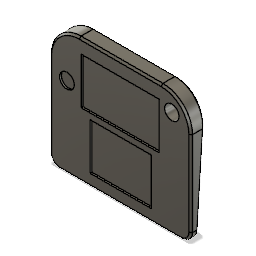
Key Chain - 2DS v1 (Autodesk Fusion 360 design; units mm, degrees)
Autodesk Fusion 360 part; units mm, degrees
note: some values were not read from the file. Set by a fixed rule: which sketch regions a step uses.
(part 1 of 2)
sketch "Sketch1" plane through (0, 0, 0) normal (0, 0, 1) x (1, 0, 0)
  line L0 (8.0698, -0.1323) -> (30.0302, -0.1323)
  arc A0 (30.0302, -0.1323) -> (37.9677, -8.0698) centre (30.0302, -8.0698) cw
  line L1 (37.9677, -8.0698) -> (37.9677, -30.824)
  arc A1 (37.9677, -30.824) -> (35.3219, -33.4698) centre (35.3219, -30.824) cw
  line L2 (35.3219, -33.4698) -> (2.7781, -33.4698)
  arc A2 (2.7781, -33.4698) -> (0.1323, -30.824) centre (2.7781, -30.824) cw
  line L3 (0.1323, -30.824) -> (0.1323, -8.0698)
  arc A3 (0.1323, -8.0698) -> (8.0698, -0.1323) centre (8.0698, -8.0698) cw
  line L4 (8.599, -3.8365) -> (29.501, -3.8365)
  line L5 (29.501, -3.8365) -> (29.501, -16.2719)
  line L6 (29.501, -16.2719) -> (8.599, -16.2719)
  line L7 (8.599, -16.2719) -> (8.599, -3.8365)
  circle A4 centre (4.7625, -11.9063) radius 1.9844
  line L8 (10.9802, -17.8594) -> (27.3844, -17.8594)
  line L9 (27.3844, -17.8594) -> (27.3844, -30.2948)
  line L10 (27.3844, -30.2948) -> (10.9802, -30.2948)
  line L11 (10.9802, -30.2948) -> (10.9802, -17.8594)
  point P0 (6.7469, -11.9063)
extrude "Extrude1" add sketch "Sketch1" along normal blind 2
extrude "Extrude2" add sketch "Sketch1" along normal blind 0.5 contours L4 L5 L6 L7 | A4 | L8 L9 L10 L11
scale "Scale1" factor 1.030792 about (37.9677, -8.0698, 2) bodies 1
draft "Draft1" angle 3.8 neutral plane through (35.2404, -34.2519, -0.0616) pull (0, -1, 0) 1 faces at (22.2403, -22.7972, -0.0616)
extrude "Extrude3" add 3 faces at (14.8765, -7.9789, 0.4538) (3.8617, -11.4913, 0.4538) (15.7856, -22.4336, 0.4538) along direction (0, 0, 1) blind 1.046
sketch "Sketch2" plane through (0, 0, 2) normal (0, 0, 1) x (1, 0, 0)
  circle A0 centre (3.7401, -12.0244) radius 2.0455
  line L0 (27.0585, -30.9791) -> (10.1492, -30.9791)
  line L1 (10.1492, -30.9791) -> (10.1492, -18.1608)
  line L2 (10.1492, -18.1608) -> (27.0585, -18.1608)
  line L3 (27.0585, -18.1608) -> (27.0585, -30.9791)
  line L4 (29.2403, -16.5244) -> (7.6946, -16.5244)
  line L5 (7.6946, -16.5244) -> (7.6946, -3.7061)
  line L6 (7.6946, -3.7061) -> (29.2403, -3.7061)
  line L7 (29.2403, -3.7061) -> (29.2403, -16.5244)
  line L8 (-1.0327, -8.0698) -> (-1.0327, -31.5246)
  arc A1 (-1.0327, -31.5246) -> (1.6946, -34.2519) centre (1.6946, -31.5246) ccw
  line L9 (1.6946, -34.2519) -> (35.2404, -34.2519)
  arc A2 (35.2404, -34.2519) -> (37.9677, -31.5246) centre (35.2404, -31.5246) ccw
  line L10 (37.9677, -31.5246) -> (37.9677, -8.0698)
  arc A3 (37.9677, -8.0698) -> (29.7858, 0.1121) centre (29.7858, -8.0698) ccw
  line L11 (29.7858, 0.1121) -> (7.1492, 0.1121)
  arc A4 (7.1492, 0.1121) -> (-1.0327, -8.0698) centre (7.1492, -8.0698) ccw
  line L12 (35.5713, -2.2843) -> (29.7858, -8.0698)
  line L13 (29.7858, -8.0698) -> (35.5713, -2.2843)
  line L14 (35.5713, -2.2843) -> (34.1571, -3.6985)
  circle A5 centre (32.7429, -5.1127) radius 2
  dimension "d10" = 2
  dimension "d11" = 4
  constraint midpoint A3 L12.start
  constraint coincident A3.centre L12.end
  constraint parallel L12 L13
  constraint parallel L13 L14
  constraint coincident L14.end A5
  measures "d10" distance of L12.start L14.end
  measures "d11" diameter of A5
extrude "Extrude4" cut sketch "Sketch2" against normal blind 27 contours L12 L13 A5 | L12 L13 A5
chamfer "Chamfer1" distance 0.5 angle 45 8 edges at (1.3637, -2.2843, 2) (-1.0327, -19.7972, 2) (-0.2339, -33.4531, 2) (18.4675, -34.2519, 2) (37.1689, -33.4531, 2) (37.9677, -19.7972, 2) (35.5713, -2.2843, 2) (18.4675, 0.1121, 2)
chamfer "Chamfer2" distance 0.5 angle 45 8 edges at (37.1689, -33.4531, -0.1146) (18.4675, -34.2519, -0.0616) (-0.2339, -33.4531, -0.1146) (-1.0327, -19.7972, -1.0217) (1.3637, -2.2843, -2.1849) (18.4675, 0.1121, -2.344) (35.5713, -2.2843, -2.1849) (37.9677, -19.7972, -1.0217)
sketch "Sketch3" plane through (0, -0.1545, -2.3263) normal (0, -0.066274, -0.997801) x (-1, 0, 0)
  ellipse E0 centre (-32.7429, -4.9691) end of major axis (-32.7429, -6.9736) minor radius 2
  spline S0 degree 3 poles (-7.1492, -0.2328) (-5.9064, -0.2328) (-4.6648, -0.5408) (-2.8861, -1.4812) (-2.2609, -1.9432) (-1.7176, -2.4877) (-1.1744, -3.0321) (-0.7133, -3.6587) (-0.0624, -4.8954) (0.1618, -5.487) (0.4582, -6.6971) (0.5327, -7.3149) (0.5327, -7.9327) knots -3.141593 -3.141593 -3.141593 -3.141593 -2.656195 -2.656195 -2.356194 -2.356194 -2.356194 -2.056194 -2.056194 -1.81147 -1.81147 -1.570796 -1.570796 -1.570796 -1.570796
  line L0 (-7.1492, -0.2328) -> (-29.7858, -0.2328)
  spline S1 degree 3 poles (-37.4677, -7.9327) (-37.4677, -6.6867) (-37.1602, -5.4418) (-36.2217, -3.6587) (-35.7606, -3.0321) (-35.2173, -2.4877) (-34.6741, -1.9432) (-34.0489, -1.4812) (-32.8198, -0.8314) (-32.2349, -0.608) (-31.0285, -0.3087) (-30.4072, -0.2328) (-29.7858, -0.2328) knots -1.570796 -1.570796 -1.570796 -1.570796 -1.085399 -1.085399 -0.785398 -0.785398 -0.785398 -0.485397 -0.485397 -0.242699 -0.242699 0 0 0 0
  line L1 (-37.4677, -7.9659) -> (-37.4677, -7.9327)
  line L2 (-37.4677, -7.9659) -> (-37.4677, -31.4392)
  spline S2 degree 3 poles (-37.4675, -31.4663) (-37.4676, -31.4618) (-37.4676, -31.4573) (-37.4677, -31.4482) (-37.4677, -31.4437) (-37.4677, -31.4392) knots -1.582946 -1.582946 -1.582946 -1.582946 -1.576871 -1.576871 -1.570796 -1.570796 -1.570796 -1.570796
  spline S3 degree 3 poles (-35.2404, -33.6725) (-35.6025, -33.6725) (-35.9643, -33.5823) (-36.4792, -33.3084) (-36.6588, -33.1753) (-36.815, -33.0188) (-36.9712, -32.8622) (-37.104, -32.6822) (-37.3733, -32.1737) (-37.4632, -31.8207) (-37.4675, -31.4663) knots -3.141593 -3.141593 -3.141593 -3.141593 -2.653648 -2.653648 -2.356194 -2.356194 -2.356194 -2.058741 -2.058741 -1.582946 -1.582946 -1.582946 -1.582946
  line L3 (-35.2404, -33.6725) -> (-1.6946, -33.6725)
  spline S4 degree 3 poles (0.5326, -31.4663) (0.5283, -31.8207) (0.4383, -32.1737) (0.169, -32.6822) (0.0362, -32.8622) (-0.12, -33.0188) (-0.2762, -33.1753) (-0.4558, -33.3084) (-0.9707, -33.5823) (-1.3325, -33.6725) (-1.6946, -33.6725) knots -1.558647 -1.558647 -1.558647 -1.558647 -1.082852 -1.082852 -0.785398 -0.785398 -0.785398 -0.487945 -0.487945 0 0 0 0
  spline S5 degree 3 poles (0.5327, -31.4392) (0.5327, -31.4437) (0.5327, -31.4482) (0.5327, -31.4573) (0.5326, -31.4618) (0.5326, -31.4663) knots -1.570796 -1.570796 -1.570796 -1.570796 -1.564722 -1.564722 -1.558647 -1.558647 -1.558647 -1.558647
  line L4 (0.5327, -31.4392) -> (0.5327, -7.9659)
  line L5 (0.5327, -7.9327) -> (0.5327, -7.9659)
  line L6 (-28.5549, -9.3081) -> (-28.5549, -9.5789)
  line L7 (-28.5549, -9.5789) -> (-28.8258, -9.5789)
  line L8 (-28.8258, -9.5789) -> (-28.8258, -9.8498)
  line L9 (-28.8258, -9.8498) -> (-29.0966, -9.8498)
  line L10 (-29.0966, -9.8498) -> (-29.0966, -10.1206)
  line L11 (-29.0966, -10.1206) -> (-29.3674, -10.1206)
  line L12 (-29.3674, -10.1206) -> (-29.3674, -10.3914)
  line L13 (-29.3674, -10.3914) -> (-29.6383, -10.3914)
  line L14 (-29.6383, -10.3914) -> (-29.6383, -10.6623)
  line L15 (-29.6383, -10.6623) -> (-29.9091, -10.6623)
  line L16 (-29.9091, -10.6623) -> (-29.9091, -11.2039)
  line L17 (-29.9091, -11.2039) -> (-28.2841, -11.2039)
  line L18 (-28.2841, -11.2039) -> (-28.2841, -15.2664)
  line L19 (-28.2841, -15.2664) -> (-29.9091, -15.2664)
  line L20 (-29.9091, -15.2664) -> (-29.9091, -16.6206)
  line L21 (-29.9091, -16.6206) -> (-25.8466, -16.6206)
  line L22 (-25.8466, -16.6206) -> (-25.8466, -15.2664)
  line L23 (-25.8466, -15.2664) -> (-26.9299, -15.2664)
  line L24 (-26.9299, -15.2664) -> (-26.9299, -9.3081)
  line L25 (-26.9299, -9.3081) -> (-28.5549, -9.3081)
  line L26 (-24.2216, -9.3081) -> (-24.2216, -9.5789)
  line L27 (-24.2216, -9.5789) -> (-24.4924, -9.5789)
  line L28 (-24.4924, -9.5789) -> (-24.4924, -9.8498)
  line L29 (-24.4924, -9.8498) -> (-24.7633, -9.8498)
  line L30 (-24.7633, -9.8498) -> (-24.7633, -10.1206)
  line L31 (-24.7633, -10.1206) -> (-25.0341, -10.1206)
  line L32 (-25.0341, -10.1206) -> (-25.0341, -10.3914)
  line L33 (-25.0341, -10.3914) -> (-25.3049, -10.3914)
  line L34 (-25.3049, -10.3914) -> (-25.3049, -15.5373)
  line L35 (-25.3049, -15.5373) -> (-25.0341, -15.5373)
  line L36 (-25.0341, -15.5373) -> (-25.0341, -15.8081)
  line L37 (-25.0341, -15.8081) -> (-24.7633, -15.8081)
  line L38 (-24.7633, -15.8081) -> (-24.7633, -16.0789)
  line L39 (-24.7633, -16.0789) -> (-24.4924, -16.0789)
  line L40 (-24.4924, -16.0789) -> (-24.4924, -16.3498)
  line L41 (-24.4924, -16.3498) -> (-24.2216, -16.3498)
  line L42 (-24.2216, -16.3498) -> (-24.2216, -16.6206)
  line L43 (-24.2216, -16.6206) -> (-21.7841, -16.6206)
  line L44 (-21.7841, -16.6206) -> (-21.7841, -16.3498)
  line L45 (-21.7841, -16.3498) -> (-21.5133, -16.3498)
  line L46 (-21.5133, -16.3498) -> (-21.5133, -16.0789)
  line L47 (-21.5133, -16.0789) -> (-21.2424, -16.0789)
  line L48 (-21.2424, -16.0789) -> (-21.2424, -15.8081)
  line L49 (-21.2424, -15.8081) -> (-20.9716, -15.8081)
  line L50 (-20.9716, -15.8081) -> (-20.9716, -13.3706)
  line L51 (-20.9716, -13.3706) -> (-21.2424, -13.3706)
  line L52 (-21.2424, -13.3706) -> (-21.2424, -13.0998)
  line L53 (-21.2424, -13.0998) -> (-21.5133, -13.0998)
  line L54 (-21.5133, -13.0998) -> (-21.5133, -12.8289)
  line L55 (-21.5133, -12.8289) -> (-21.7841, -12.8289)
  line L56 (-21.7841, -12.8289) -> (-21.7841, -12.5581)
  line L57 (-21.7841, -12.5581) -> (-22.0549, -12.5581)
  line L58 (-22.0549, -12.5581) -> (-22.0549, -12.2873)
  line L59 (-22.0549, -12.2873) -> (-23.6799, -12.2873)
  line L60 (-23.6799, -12.2873) -> (-23.6799, -12.5581)
  line L61 (-23.6799, -12.5581) -> (-23.9508, -12.5581)
  line L62 (-23.9508, -12.5581) -> (-23.9508, -11.4748)
  line L63 (-23.9508, -11.4748) -> (-23.6799, -11.4748)
  line L64 (-23.6799, -11.4748) -> (-23.6799, -11.2039)
  line L65 (-23.6799, -11.2039) -> (-23.4091, -11.2039)
  line L66 (-23.4091, -11.2039) -> (-23.4091, -10.9331)
  line L67 (-23.4091, -10.9331) -> (-22.5966, -10.9331)
  line L68 (-22.5966, -10.9331) -> (-22.5966, -11.2039)
  line L69 (-22.5966, -11.2039) -> (-22.3258, -11.2039)
  line L70 (-22.3258, -11.2039) -> (-22.3258, -11.7456)
  line L71 (-22.3258, -11.7456) -> (-20.9716, -11.7456)
  line L72 (-20.9716, -11.7456) -> (-20.9716, -10.3914)
  line L73 (-20.9716, -10.3914) -> (-21.2424, -10.3914)
  line L74 (-21.2424, -10.3914) -> (-21.2424, -10.1206)
  line L75 (-21.2424, -10.1206) -> (-21.5133, -10.1206)
  line L76 (-21.5133, -10.1206) -> (-21.5133, -9.8498)
  line L77 (-21.5133, -9.8498) -> (-21.7841, -9.8498)
  line L78 (-21.7841, -9.8498) -> (-21.7841, -9.5789)
  line L79 (-21.7841, -9.5789) -> (-22.0549, -9.5789)
  line L80 (-22.0549, -9.5789) -> (-22.0549, -9.3081)
  line L81 (-22.0549, -9.3081) -> (-24.2216, -9.3081)
  line L82 (-19.3466, -9.3081) -> (-19.3466, -16.6206)
  line L83 (-19.3466, -16.6206) -> (-16.9091, -16.6206)
  line L84 (-16.9091, -16.6206) -> (-16.9091, -16.3498)
  line L85 (-16.9091, -16.3498) -> (-16.6383, -16.3498)
  line L86 (-16.6383, -16.3498) -> (-16.6383, -16.0789)
  line L87 (-16.6383, -16.0789) -> (-16.3674, -16.0789)
  line L88 (-16.3674, -16.0789) -> (-16.3674, -15.8081)
  line L89 (-16.3674, -15.8081) -> (-16.0966, -15.8081)
  line L90 (-16.0966, -15.8081) -> (-16.0966, -13.3706)
  line L91 (-16.0966, -13.3706) -> (-16.3674, -13.3706)
  line L92 (-16.3674, -13.3706) -> (-16.3674, -13.0998)
  line L93 (-16.3674, -13.0998) -> (-16.6383, -13.0998)
  line L94 (-16.6383, -13.0998) -> (-16.6383, -12.8289)
  line L95 (-16.6383, -12.8289) -> (-16.3674, -12.8289)
  line L96 (-16.3674, -12.8289) -> (-16.3674, -12.5581)
  line L97 (-16.3674, -12.5581) -> (-16.0966, -12.5581)
  line L98 (-16.0966, -12.5581) -> (-16.0966, -10.1206)
  line L99 (-16.0966, -10.1206) -> (-16.3674, -10.1206)
  line L100 (-16.3674, -10.1206) -> (-16.3674, -9.8498)
  line L101 (-16.3674, -9.8498) -> (-16.6383, -9.8498)
  line L102 (-16.6383, -9.8498) -> (-16.6383, -9.5789)
  line L103 (-16.6383, -9.5789) -> (-16.9091, -9.5789)
  line L104 (-16.9091, -9.5789) -> (-16.9091, -9.3081)
  line L105 (-16.9091, -9.3081) -> (-19.3466, -9.3081)
  line L106 (-15.5549, -9.3081) -> (-15.5549, -10.6623)
  line L107 (-15.5549, -10.6623) -> (-14.4716, -10.6623)
  line L108 (-14.4716, -10.6623) -> (-14.4716, -15.2664)
  line L109 (-14.4716, -15.2664) -> (-15.5549, -15.2664)
  line L110 (-15.5549, -15.2664) -> (-15.5549, -16.6206)
  line L111 (-15.5549, -16.6206) -> (-11.7633, -16.6206)
  line L112 (-11.7633, -16.6206) -> (-11.7633, -15.2664)
  line L113 (-11.7633, -15.2664) -> (-12.8466, -15.2664)
  line L114 (-12.8466, -15.2664) -> (-12.8466, -10.6623)
  line L115 (-12.8466, -10.6623) -> (-11.7633, -10.6623)
  line L116 (-11.7633, -10.6623) -> (-11.7633, -9.3081)
  line L117 (-11.7633, -9.3081) -> (-15.5549, -9.3081)
  line L118 (-11.2216, -9.3081) -> (-11.2216, -10.6623)
  line L119 (-11.2216, -10.6623) -> (-10.1383, -10.6623)
  line L120 (-10.1383, -10.6623) -> (-10.1383, -16.6206)
  line L121 (-10.1383, -16.6206) -> (-8.5133, -16.6206)
  line L122 (-8.5133, -16.6206) -> (-8.5133, -10.6623)
  line L123 (-8.5133, -10.6623) -> (-7.4299, -10.6623)
  line L124 (-7.4299, -10.6623) -> (-7.4299, -9.3081)
  line L125 (-7.4299, -9.3081) -> (-11.2216, -9.3081)
  line L126 (-27.2008, -9.5789) -> (-27.2008, -15.5373)
  line L127 (-27.2008, -15.5373) -> (-26.1174, -15.5373)
  line L128 (-26.1174, -15.5373) -> (-26.1174, -16.3498)
  line L129 (-26.1174, -16.3498) -> (-29.6383, -16.3498)
  line L130 (-29.6383, -16.3498) -> (-29.6383, -15.5373)
  line L131 (-29.6383, -15.5373) -> (-28.0133, -15.5373)
  line L132 (-28.0133, -15.5373) -> (-28.0133, -10.9331)
  line L133 (-28.0133, -10.9331) -> (-29.3674, -10.9331)
  line L134 (-29.3674, -10.9331) -> (-29.3674, -10.6623)
  line L135 (-29.3674, -10.6623) -> (-29.0966, -10.6623)
  line L136 (-29.0966, -10.6623) -> (-29.0966, -10.3914)
  line L137 (-29.0966, -10.3914) -> (-28.8258, -10.3914)
  line L138 (-28.8258, -10.3914) -> (-28.8258, -10.1206)
  line L139 (-28.8258, -10.1206) -> (-28.5549, -10.1206)
  line L140 (-28.5549, -10.1206) -> (-28.5549, -9.8498)
  line L141 (-28.5549, -9.8498) -> (-28.2841, -9.8498)
  line L142 (-28.2841, -9.8498) -> (-28.2841, -9.5789)
  line L143 (-28.2841, -9.5789) -> (-27.2008, -9.5789)
  line L144 (-22.3258, -9.5789) -> (-22.3258, -9.8498)
  line L145 (-22.3258, -9.8498) -> (-22.0549, -9.8498)
  line L146 (-22.0549, -9.8498) -> (-22.0549, -10.1206)
  line L147 (-22.0549, -10.1206) -> (-21.7841, -10.1206)
  line L148 (-21.7841, -10.1206) -> (-21.7841, -10.3914)
  line L149 (-21.7841, -10.3914) -> (-21.5133, -10.3914)
  line L150 (-21.5133, -10.3914) -> (-21.5133, -10.6623)
  line L151 (-21.5133, -10.6623) -> (-21.2424, -10.6623)
  line L152 (-21.2424, -10.6623) -> (-21.2424, -11.4748)
  line L153 (-21.2424, -11.4748) -> (-22.0549, -11.4748)
  line L154 (-22.0549, -11.4748) -> (-22.0549, -10.9331)
  line L155 (-22.0549, -10.9331) -> (-22.3258, -10.9331)
  line L156 (-22.3258, -10.9331) -> (-22.3258, -10.6623)
  line L157 (-22.3258, -10.6623) -> (-23.6799, -10.6623)
  line L158 (-23.6799, -10.6623) -> (-23.6799, -10.9331)
  line L159 (-23.6799, -10.9331) -> (-23.9508, -10.9331)
  line L160 (-23.9508, -10.9331) -> (-23.9508, -11.2039)
  line L161 (-23.9508, -11.2039) -> (-24.2216, -11.2039)
  line L162 (-24.2216, -11.2039) -> (-24.2216, -13.0998)
  line L163 (-24.2216, -13.0998) -> (-23.6799, -13.0998)
  line L164 (-23.6799, -13.0998) -> (-23.6799, -12.8289)
  line L165 (-23.6799, -12.8289) -> (-23.4091, -12.8289)
  line L166 (-23.4091, -12.8289) -> (-23.4091, -12.5581)
  line L167 (-23.4091, -12.5581) -> (-22.3258, -12.5581)
  line L168 (-22.3258, -12.5581) -> (-22.3258, -12.8289)
  line L169 (-22.3258, -12.8289) -> (-22.0549, -12.8289)
  line L170 (-22.0549, -12.8289) -> (-22.0549, -13.0998)
  line L171 (-22.0549, -13.0998) -> (-21.7841, -13.0998)
  line L172 (-21.7841, -13.0998) -> (-21.7841, -13.3706)
  line L173 (-21.7841, -13.3706) -> (-21.5133, -13.3706)
  line L174 (-21.5133, -13.3706) -> (-21.5133, -13.6414)
  line L175 (-21.5133, -13.6414) -> (-21.2424, -13.6414)
  line L176 (-21.2424, -13.6414) -> (-21.2424, -15.5373)
  line L177 (-21.2424, -15.5373) -> (-21.5133, -15.5373)
  line L178 (-21.5133, -15.5373) -> (-21.5133, -15.8081)
  line L179 (-21.5133, -15.8081) -> (-21.7841, -15.8081)
  line L180 (-21.7841, -15.8081) -> (-21.7841, -16.0789)
  line L181 (-21.7841, -16.0789) -> (-22.0549, -16.0789)
  line L182 (-22.0549, -16.0789) -> (-22.0549, -16.3498)
  line L183 (-22.0549, -16.3498) -> (-23.9508, -16.3498)
  line L184 (-23.9508, -16.3498) -> (-23.9508, -16.0789)
  line L185 (-23.9508, -16.0789) -> (-24.2216, -16.0789)
  line L186 (-24.2216, -16.0789) -> (-24.2216, -15.8081)
  line L187 (-24.2216, -15.8081) -> (-24.4924, -15.8081)
  line L188 (-24.4924, -15.8081) -> (-24.4924, -15.5373)
  line L189 (-24.4924, -15.5373) -> (-24.7633, -15.5373)
  line L190 (-24.7633, -15.5373) -> (-24.7633, -15.2664)
  line L191 (-24.7633, -15.2664) -> (-25.0341, -15.2664)
  line L192 (-25.0341, -15.2664) -> (-25.0341, -10.6623)
  line L193 (-25.0341, -10.6623) -> (-24.7633, -10.6623)
  line L194 (-24.7633, -10.6623) -> (-24.7633, -10.3914)
  line L195 (-24.7633, -10.3914) -> (-24.4924, -10.3914)
  line L196 (-24.4924, -10.3914) -> (-24.4924, -10.1206)
  line L197 (-24.4924, -10.1206) -> (-24.2216, -10.1206)
  line L198 (-24.2216, -10.1206) -> (-24.2216, -9.8498)
  line L199 (-24.2216, -9.8498) -> (-23.9508, -9.8498)
  line L200 (-23.9508, -9.8498) -> (-23.9508, -9.5789)
  line L201 (-23.9508, -9.5789) -> (-22.3258, -9.5789)
  line L202 (-17.1799, -9.5789) -> (-17.1799, -9.8498)
  line L203 (-17.1799, -9.8498) -> (-16.9091, -9.8498)
  line L204 (-16.9091, -9.8498) -> (-16.9091, -10.1206)
  line L205 (-16.9091, -10.1206) -> (-16.6383, -10.1206)
  line L206 (-16.6383, -10.1206) -> (-16.6383, -10.3914)
  line L207 (-16.6383, -10.3914) -> (-16.3674, -10.3914)
  line L208 (-16.3674, -10.3914) -> (-16.3674, -12.2873)
  line L209 (-16.3674, -12.2873) -> (-16.6383, -12.2873)
  line L210 (-16.6383, -12.2873) -> (-16.6383, -12.5581)
  line L211 (-16.6383, -12.5581) -> (-17.4508, -12.5581)
  line L212 (-17.4508, -12.5581) -> (-17.4508, -12.8289)
  line L213 (-17.4508, -12.8289) -> (-17.1799, -12.8289)
  line L214 (-17.1799, -12.8289) -> (-17.1799, -13.0998)
  line L215 (-17.1799, -13.0998) -> (-16.9091, -13.0998)
  line L216 (-16.9091, -13.0998) -> (-16.9091, -13.3706)
  line L217 (-16.9091, -13.3706) -> (-16.6383, -13.3706)
  line L218 (-16.6383, -13.3706) -> (-16.6383, -13.6414)
  line L219 (-16.6383, -13.6414) -> (-16.3674, -13.6414)
  line L220 (-16.3674, -13.6414) -> (-16.3674, -15.5373)
  line L221 (-16.3674, -15.5373) -> (-16.6383, -15.5373)
  line L222 (-16.6383, -15.5373) -> (-16.6383, -15.8081)
  line L223 (-16.6383, -15.8081) -> (-16.9091, -15.8081)
  line L224 (-16.9091, -15.8081) -> (-16.9091, -16.0789)
  line L225 (-16.9091, -16.0789) -> (-17.1799, -16.0789)
  line L226 (-17.1799, -16.0789) -> (-17.1799, -16.3498)
  line L227 (-17.1799, -16.3498) -> (-19.0758, -16.3498)
  line L228 (-19.0758, -16.3498) -> (-19.0758, -9.5789)
  line L229 (-19.0758, -9.5789) -> (-17.1799, -9.5789)
  line L230 (-12.0341, -9.5789) -> (-12.0341, -10.3914)
  line L231 (-12.0341, -10.3914) -> (-13.1174, -10.3914)
  line L232 (-13.1174, -10.3914) -> (-13.1174, -15.5373)
  line L233 (-13.1174, -15.5373) -> (-12.0341, -15.5373)
  line L234 (-12.0341, -15.5373) -> (-12.0341, -16.3498)
  line L235 (-12.0341, -16.3498) -> (-15.2841, -16.3498)
  line L236 (-15.2841, -16.3498) -> (-15.2841, -15.5373)
  line L237 (-15.2841, -15.5373) -> (-14.2008, -15.5373)
  line L238 (-14.2008, -15.5373) -> (-14.2008, -10.3914)
  line L239 (-14.2008, -10.3914) -> (-15.2841, -10.3914)
  line L240 (-15.2841, -10.3914) -> (-15.2841, -9.5789)
  line L241 (-15.2841, -9.5789) -> (-12.0341, -9.5789)
  line L242 (-7.7008, -9.5789) -> (-7.7008, -10.3914)
  line L243 (-7.7008, -10.3914) -> (-8.7841, -10.3914)
  line L244 (-8.7841, -10.3914) -> (-8.7841, -16.3498)
  line L245 (-8.7841, -16.3498) -> (-9.8674, -16.3498)
  line L246 (-9.8674, -16.3498) -> (-9.8674, -10.3914)
  line L247 (-9.8674, -10.3914) -> (-10.9508, -10.3914)
  line L248 (-10.9508, -10.3914) -> (-10.9508, -9.5789)
  line L249 (-10.9508, -9.5789) -> (-7.7008, -9.5789)
  line L250 (-18.5341, -10.1206) -> (-18.5341, -12.0164)
  line L251 (-18.5341, -12.0164) -> (-17.4508, -12.0164)
  line L252 (-17.4508, -12.0164) -> (-17.4508, -11.7456)
  line L253 (-17.4508, -11.7456) -> (-17.1799, -11.7456)
  line L254 (-17.1799, -11.7456) -> (-17.1799, -10.3914)
  line L255 (-17.1799, -10.3914) -> (-17.4508, -10.3914)
  line L256 (-17.4508, -10.3914) -> (-17.4508, -10.1206)
  line L257 (-17.4508, -10.1206) -> (-18.5341, -10.1206)
  line L258 (-17.7216, -10.3914) -> (-17.7216, -10.6623)
  line L259 (-17.7216, -10.6623) -> (-17.4508, -10.6623)
  line L260 (-17.4508, -10.6623) -> (-17.4508, -11.4748)
  line L261 (-17.4508, -11.4748) -> (-17.7216, -11.4748)
  line L262 (-17.7216, -11.4748) -> (-17.7216, -11.7456)
  line L263 (-17.7216, -11.7456) -> (-18.2633, -11.7456)
  line L264 (-18.2633, -11.7456) -> (-18.2633, -10.3914)
  line L265 (-18.2633, -10.3914) -> (-17.7216, -10.3914)
  line L266 (-23.6799, -13.3706) -> (-23.6799, -13.6414)
  line L267 (-23.6799, -13.6414) -> (-23.9508, -13.6414)
  line L268 (-23.9508, -13.6414) -> (-23.9508, -13.9123)
  line L269 (-23.9508, -13.9123) -> (-24.2216, -13.9123)
  line L270 (-24.2216, -13.9123) -> (-24.2216, -15.2664)
  line L271 (-24.2216, -15.2664) -> (-23.9508, -15.2664)
  line L272 (-23.9508, -15.2664) -> (-23.9508, -15.5373)
  line L273 (-23.9508, -15.5373) -> (-23.6799, -15.5373)
  line L274 (-23.6799, -15.5373) -> (-23.6799, -15.8081)
  line L275 (-23.6799, -15.8081) -> (-22.5966, -15.8081)
  line L276 (-22.5966, -15.8081) -> (-22.5966, -15.5373)
  line L277 (-22.5966, -15.5373) -> (-22.3258, -15.5373)
  line L278 (-22.3258, -15.5373) -> (-22.3258, -15.2664)
  line L279 (-22.3258, -15.2664) -> (-22.0549, -15.2664)
  line L280 (-22.0549, -15.2664) -> (-22.0549, -13.9123)
  line L281 (-22.0549, -13.9123) -> (-22.3258, -13.9123)
  line L282 (-22.3258, -13.9123) -> (-22.3258, -13.6414)
  line L283 (-22.3258, -13.6414) -> (-22.5966, -13.6414)
  line L284 (-22.5966, -13.6414) -> (-22.5966, -13.3706)
  line L285 (-22.5966, -13.3706) -> (-23.6799, -13.3706)
  line L286 (-18.5341, -13.3706) -> (-18.5341, -15.5373)
  line L287 (-18.5341, -15.5373) -> (-17.4508, -15.5373)
  line L288 (-17.4508, -15.5373) -> (-17.4508, -15.2664)
  line L289 (-17.4508, -15.2664) -> (-17.1799, -15.2664)
  line L290 (-17.1799, -15.2664) -> (-17.1799, -13.6414)
  line L291 (-17.1799, -13.6414) -> (-17.4508, -13.6414)
  line L292 (-17.4508, -13.6414) -> (-17.4508, -13.3706)
  line L293 (-17.4508, -13.3706) -> (-18.5341, -13.3706)
  line L294 (-22.8674, -13.6414) -> (-22.8674, -13.9123)
  line L295 (-22.8674, -13.9123) -> (-22.5966, -13.9123)
  line L296 (-22.5966, -13.9123) -> (-22.5966, -14.1831)
  line L297 (-22.5966, -14.1831) -> (-22.3258, -14.1831)
  line L298 (-22.3258, -14.1831) -> (-22.3258, -14.9956)
  line L299 (-22.3258, -14.9956) -> (-22.5966, -14.9956)
  line L300 (-22.5966, -14.9956) -> (-22.5966, -15.2664)
  line L301 (-22.5966, -15.2664) -> (-22.8674, -15.2664)
  line L302 (-22.8674, -15.2664) -> (-22.8674, -15.5373)
  line L303 (-22.8674, -15.5373) -> (-23.4091, -15.5373)
  line L304 (-23.4091, -15.5373) -> (-23.4091, -15.2664)
  line L305 (-23.4091, -15.2664) -> (-23.6799, -15.2664)
  line L306 (-23.6799, -15.2664) -> (-23.6799, -14.9956)
  line L307 (-23.6799, -14.9956) -> (-23.9508, -14.9956)
  line L308 (-23.9508, -14.9956) -> (-23.9508, -14.1831)
  line L309 (-23.9508, -14.1831) -> (-23.6799, -14.1831)
  line L310 (-23.6799, -14.1831) -> (-23.6799, -13.9123)
  line L311 (-23.6799, -13.9123) -> (-23.4091, -13.9123)
  line L312 (-23.4091, -13.9123) -> (-23.4091, -13.6414)
  line L313 (-23.4091, -13.6414) -> (-22.8674, -13.6414)
  line L314 (-17.7216, -13.6414) -> (-17.7216, -13.9123)
  line L315 (-17.7216, -13.9123) -> (-17.4508, -13.9123)
  line L316 (-17.4508, -13.9123) -> (-17.4508, -14.9956)
  line L317 (-17.4508, -14.9956) -> (-17.7216, -14.9956)
  line L318 (-17.7216, -14.9956) -> (-17.7216, -15.2664)
  line L319 (-17.7216, -15.2664) -> (-18.2633, -15.2664)
  line L320 (-18.2633, -15.2664) -> (-18.2633, -13.6414)
  line L321 (-18.2633, -13.6414) -> (-17.7216, -13.6414)
  line L322 (-28.8258, -17.4331) -> (-28.8258, -17.7039)
  line L323 (-28.8258, -17.7039) -> (-29.0966, -17.7039)
  line L324 (-29.0966, -17.7039) -> (-29.0966, -17.9748)
  line L325 (-29.0966, -17.9748) -> (-29.3674, -17.9748)
  line L326 (-29.3674, -17.9748) -> (-29.3674, -18.2456)
  line L327 (-29.3674, -18.2456) -> (-29.6383, -18.2456)
  line L328 (-29.6383, -18.2456) -> (-29.6383, -18.5164)
  line L329 (-29.6383, -18.5164) -> (-29.9091, -18.5164)
  line L330 (-29.9091, -18.5164) -> (-29.9091, -21.2248)
  line L331 (-29.9091, -21.2248) -> (-29.6383, -21.2248)
  line L332 (-29.6383, -21.2248) -> (-29.6383, -21.4956)
  line L333 (-29.6383, -21.4956) -> (-29.3674, -21.4956)
  line L334 (-29.3674, -21.4956) -> (-29.3674, -21.7664)
  line L335 (-29.3674, -21.7664) -> (-29.0966, -21.7664)
  line L336 (-29.0966, -21.7664) -> (-29.0966, -22.0373)
  line L337 (-29.0966, -22.0373) -> (-28.8258, -22.0373)
  line L338 (-28.8258, -22.0373) -> (-28.8258, -22.3081)
  line L339 (-28.8258, -22.3081) -> (-26.9299, -22.3081)
  line L340 (-26.9299, -22.3081) -> (-26.9299, -22.0373)
  line L341 (-26.9299, -22.0373) -> (-26.6591, -22.0373)
  line L342 (-26.6591, -22.0373) -> (-26.6591, -21.7664)
  line L343 (-26.6591, -21.7664) -> (-26.3883, -21.7664)
  line L344 (-26.3883, -21.7664) -> (-26.3883, -21.4956)
  line L345 (-26.3883, -21.4956) -> (-26.1174, -21.4956)
  line L346 (-26.1174, -21.4956) -> (-26.1174, -19.3289)
  line L347 (-26.1174, -19.3289) -> (-28.0133, -19.3289)
  line L348 (-28.0133, -19.3289) -> (-28.0133, -20.4123)
  line L349 (-28.0133, -20.4123) -> (-26.9299, -20.4123)
  line L350 (-26.9299, -20.4123) -> (-26.9299, -20.6831)
  line L351 (-26.9299, -20.6831) -> (-27.2008, -20.6831)
  line L352 (-27.2008, -20.6831) -> (-27.2008, -20.9539)
  line L353 (-27.2008, -20.9539) -> (-27.4716, -20.9539)
  line L354 (-27.4716, -20.9539) -> (-27.4716, -21.2248)
  line L355 (-27.4716, -21.2248) -> (-28.2841, -21.2248)
  line L356 (-28.2841, -21.2248) -> (-28.2841, -20.9539)
  line L357 (-28.2841, -20.9539) -> (-28.5549, -20.9539)
  line L358 (-28.5549, -20.9539) -> (-28.5549, -20.6831)
  line L359 (-28.5549, -20.6831) -> (-28.8258, -20.6831)
  line L360 (-28.8258, -20.6831) -> (-28.8258, -19.0581)
  line L361 (-28.8258, -19.0581) -> (-28.5549, -19.0581)
  line L362 (-28.5549, -19.0581) -> (-28.5549, -18.7873)
  line L363 (-28.5549, -18.7873) -> (-28.2841, -18.7873)
  line L364 (-28.2841, -18.7873) -> (-28.2841, -18.5164)
  line L365 (-28.2841, -18.5164) -> (-26.9299, -18.5164)
  line L366 (-26.9299, -18.5164) -> (-26.9299, -17.4331)
  line L367 (-26.9299, -17.4331) -> (-28.8258, -17.4331)
  line L368 (-23.9508, -17.4331) -> (-23.9508, -17.7039)
  line L369 (-23.9508, -17.7039) -> (-24.2216, -17.7039)
  line L370 (-24.2216, -17.7039) -> (-24.2216, -17.9748)
  line L371 (-24.2216, -17.9748) -> (-24.4924, -17.9748)
  line L372 (-24.4924, -17.9748) -> (-24.4924, -18.2456)
  line L373 (-24.4924, -18.2456) -> (-24.7633, -18.2456)
  line L374 (-24.7633, -18.2456) -> (-24.7633, -18.5164)
  line L375 (-24.7633, -18.5164) -> (-25.0341, -18.5164)
  line L376 (-25.0341, -18.5164) -> (-25.0341, -22.3081)
  line L377 (-25.0341, -22.3081) -> (-23.9508, -22.3081)
  line L378 (-23.9508, -22.3081) -> (-23.9508, -21.2248)
  line L379 (-23.9508, -21.2248) -> (-23.1383, -21.2248)
  line L380 (-23.1383, -21.2248) -> (-23.1383, -22.3081)
  line L381 (-23.1383, -22.3081) -> (-22.0549, -22.3081)
  line L382 (-22.0549, -22.3081) -> (-22.0549, -18.5164)
  line L383 (-22.0549, -18.5164) -> (-22.3258, -18.5164)
  line L384 (-22.3258, -18.5164) -> (-22.3258, -18.2456)
  line L385 (-22.3258, -18.2456) -> (-22.5966, -18.2456)
  line L386 (-22.5966, -18.2456) -> (-22.5966, -17.9748)
  line L387 (-22.5966, -17.9748) -> (-22.8674, -17.9748)
  line L388 (-22.8674, -17.9748) -> (-22.8674, -17.7039)
  line L389 (-22.8674, -17.7039) -> (-23.1383, -17.7039)
  line L390 (-23.1383, -17.7039) -> (-23.1383, -17.4331)
  line L391 (-23.1383, -17.4331) -> (-23.9508, -17.4331)
  line L392 (-20.1591, -17.4331) -> (-20.1591, -17.7039)
  line L393 (-20.1591, -17.7039) -> (-20.4299, -17.7039)
  line L394 (-20.4299, -17.7039) -> (-20.4299, -17.9748)
  line L395 (-20.4299, -17.9748) -> (-20.7008, -17.9748)
  line L396 (-20.7008, -17.9748) -> (-20.7008, -18.2456)
  line L397 (-20.7008, -18.2456) -> (-20.9716, -18.2456)
  line L398 (-20.9716, -18.2456) -> (-20.9716, -18.5164)
  line L399 (-20.9716, -18.5164) -> (-21.2424, -18.5164)
  line L400 (-21.2424, -18.5164) -> (-21.2424, -22.3081)
  line L401 (-21.2424, -22.3081) -> (-20.1591, -22.3081)
  line L402 (-20.1591, -22.3081) -> (-20.1591, -19.0581)
  line L403 (-20.1591, -19.0581) -> (-19.8883, -19.0581)
  line L404 (-19.8883, -19.0581) -> (-19.8883, -18.7873)
  line L405 (-19.8883, -18.7873) -> (-19.3466, -18.7873)
  line L406 (-19.3466, -18.7873) -> (-19.3466, -19.0581)
  line L407 (-19.3466, -19.0581) -> (-19.0758, -19.0581)
  line L408 (-19.0758, -19.0581) -> (-19.0758, -20.4123)
  line L409 (-19.0758, -20.4123) -> (-18.2633, -20.4123)
  line L410 (-18.2633, -20.4123) -> (-18.2633, -19.0581)
  line L411 (-18.2633, -19.0581) -> (-17.9924, -19.0581)
  line L412 (-17.9924, -19.0581) -> (-17.9924, -18.7873)
  line L413 (-17.9924, -18.7873) -> (-17.4508, -18.7873)
  line L414 (-17.4508, -18.7873) -> (-17.4508, -19.0581)
  line L415 (-17.4508, -19.0581) -> (-17.1799, -19.0581)
  line L416 (-17.1799, -19.0581) -> (-17.1799, -22.3081)
  line L417 (-17.1799, -22.3081) -> (-16.0966, -22.3081)
  line L418 (-16.0966, -22.3081) -> (-16.0966, -18.5164)
  line L419 (-16.0966, -18.5164) -> (-16.3674, -18.5164)
  line L420 (-16.3674, -18.5164) -> (-16.3674, -18.2456)
  line L421 (-16.3674, -18.2456) -> (-16.6383, -18.2456)
  line L422 (-16.6383, -18.2456) -> (-16.6383, -17.9748)
  line L423 (-16.6383, -17.9748) -> (-16.9091, -17.9748)
  line L424 (-16.9091, -17.9748) -> (-16.9091, -17.7039)
  line L425 (-16.9091, -17.7039) -> (-17.1799, -17.7039)
  line L426 (-17.1799, -17.7039) -> (-17.1799, -17.4331)
  line L427 (-17.1799, -17.4331) -> (-18.2633, -17.4331)
  line L428 (-18.2633, -17.4331) -> (-18.2633, -17.7039)
  line L429 (-18.2633, -17.7039) -> (-18.5341, -17.7039)
  line L430 (-18.5341, -17.7039) -> (-18.5341, -17.9748)
  line L431 (-18.5341, -17.9748) -> (-18.8049, -17.9748)
  line L432 (-18.8049, -17.9748) -> (-18.8049, -17.7039)
  line L433 (-18.8049, -17.7039) -> (-19.0758, -17.7039)
  line L434 (-19.0758, -17.7039) -> (-19.0758, -17.4331)
  line L435 (-19.0758, -17.4331) -> (-20.1591, -17.4331)
  line L436 (-15.2841, -17.4331) -> (-15.2841, -22.3081)
  line L437 (-15.2841, -22.3081) -> (-12.3049, -22.3081)
  line L438 (-12.3049, -22.3081) -> (-12.3049, -21.2248)
  line L439 (-12.3049, -21.2248) -> (-14.2008, -21.2248)
  line L440 (-14.2008, -21.2248) -> (-14.2008, -20.4123)
  line L441 (-14.2008, -20.4123) -> (-13.3883, -20.4123)
  line L442 (-13.3883, -20.4123) -> (-13.3883, -19.3289)
  line L443 (-13.3883, -19.3289) -> (-14.2008, -19.3289)
  line L444 (-14.2008, -19.3289) -> (-14.2008, -18.5164)
  line L445 (-14.2008, -18.5164) -> (-12.3049, -18.5164)
  line L446 (-12.3049, -18.5164) -> (-12.3049, -17.4331)
  line L447 (-12.3049, -17.4331) -> (-15.2841, -17.4331)
  line L448 (-10.4091, -17.4331) -> (-10.4091, -17.7039)
  line L449 (-10.4091, -17.7039) -> (-10.6799, -17.7039)
  line L450 (-10.6799, -17.7039) -> (-10.6799, -17.9748)
  line L451 (-10.6799, -17.9748) -> (-10.9508, -17.9748)
  line L452 (-10.9508, -17.9748) -> (-10.9508, -18.2456)
  line L453 (-10.9508, -18.2456) -> (-11.2216, -18.2456)
  line L454 (-11.2216, -18.2456) -> (-11.2216, -19.3289)
  line L455 (-11.2216, -19.3289) -> (-10.9508, -19.3289)
  line L456 (-10.9508, -19.3289) -> (-10.9508, -19.5998)
  line L457 (-10.9508, -19.5998) -> (-10.6799, -19.5998)
  line L458 (-10.6799, -19.5998) -> (-10.6799, -19.8706)
  line L459 (-10.6799, -19.8706) -> (-10.4091, -19.8706)
  line L460 (-10.4091, -19.8706) -> (-10.4091, -20.1414)
  line L461 (-10.4091, -20.1414) -> (-10.1383, -20.1414)
  line L462 (-10.1383, -20.1414) -> (-10.1383, -20.4123)
  line L463 (-10.1383, -20.4123) -> (-9.0549, -20.4123)
  line L464 (-9.0549, -20.4123) -> (-9.0549, -20.6831)
  line L465 (-9.0549, -20.6831) -> (-8.7841, -20.6831)
  line L466 (-8.7841, -20.6831) -> (-8.7841, -21.2248)
  line L467 (-8.7841, -21.2248) -> (-11.2216, -21.2248)
  line L468 (-11.2216, -21.2248) -> (-11.2216, -22.3081)
  line L469 (-11.2216, -22.3081) -> (-8.2424, -22.3081)
  line L470 (-8.2424, -22.3081) -> (-8.2424, -22.0373)
  line L471 (-8.2424, -22.0373) -> (-7.9716, -22.0373)
  line L472 (-7.9716, -22.0373) -> (-7.9716, -21.7664)
  line L473 (-7.9716, -21.7664) -> (-7.7008, -21.7664)
  line L474 (-7.7008, -21.7664) -> (-7.7008, -21.4956)
  line L475 (-7.7008, -21.4956) -> (-7.4299, -21.4956)
  line L476 (-7.4299, -21.4956) -> (-7.4299, -20.4123)
  line L477 (-7.4299, -20.4123) -> (-7.7008, -20.4123)
  line L478 (-7.7008, -20.4123) -> (-7.7008, -20.1414)
  line L479 (-7.7008, -20.1414) -> (-7.9716, -20.1414)
  line L480 (-7.9716, -20.1414) -> (-7.9716, -19.8706)
  line L481 (-7.9716, -19.8706) -> (-8.2424, -19.8706)
  line L482 (-8.2424, -19.8706) -> (-8.2424, -19.5998)
  line L483 (-8.2424, -19.5998) -> (-8.5133, -19.5998)
  line L484 (-8.5133, -19.5998) -> (-8.5133, -19.3289)
  line L485 (-8.5133, -19.3289) -> (-9.5966, -19.3289)
  line L486 (-9.5966, -19.3289) -> (-9.5966, -19.0581)
  line L487 (-9.5966, -19.0581) -> (-9.8674, -19.0581)
  line L488 (-9.8674, -19.0581) -> (-9.8674, -18.5164)
  line L489 (-9.8674, -18.5164) -> (-7.4299, -18.5164)
  line L490 (-7.4299, -18.5164) -> (-7.4299, -17.4331)
  line L491 (-7.4299, -17.4331) -> (-10.4091, -17.4331)
  line L492 (-27.2008, -17.7039) -> (-27.2008, -18.2456)
  line L493 (-27.2008, -18.2456) -> (-28.5549, -18.2456)
  line L494 (-28.5549, -18.2456) -> (-28.5549, -18.5164)
  line L495 (-28.5549, -18.5164) -> (-28.8258, -18.5164)
  line L496 (-28.8258, -18.5164) -> (-28.8258, -18.7873)
  line L497 (-28.8258, -18.7873) -> (-29.0966, -18.7873)
  line L498 (-29.0966, -18.7873) -> (-29.0966, -20.9539)
  line L499 (-29.0966, -20.9539) -> (-28.8258, -20.9539)
  line L500 (-28.8258, -20.9539) -> (-28.8258, -21.2248)
  line L501 (-28.8258, -21.2248) -> (-28.5549, -21.2248)
  line L502 (-28.5549, -21.2248) -> (-28.5549, -21.4956)
  line L503 (-28.5549, -21.4956) -> (-27.2008, -21.4956)
  line L504 (-27.2008, -21.4956) -> (-27.2008, -21.2248)
  line L505 (-27.2008, -21.2248) -> (-26.9299, -21.2248)
  line L506 (-26.9299, -21.2248) -> (-26.9299, -20.9539)
  line L507 (-26.9299, -20.9539) -> (-26.6591, -20.9539)
  line L508 (-26.6591, -20.9539) -> (-26.6591, -20.1414)
  line L509 (-26.6591, -20.1414) -> (-27.7424, -20.1414)
  line L510 (-27.7424, -20.1414) -> (-27.7424, -19.5998)
  line L511 (-27.7424, -19.5998) -> (-26.3883, -19.5998)
  line L512 (-26.3883, -19.5998) -> (-26.3883, -21.2248)
  line L513 (-26.3883, -21.2248) -> (-26.6591, -21.2248)
  line L514 (-26.6591, -21.2248) -> (-26.6591, -21.4956)
  line L515 (-26.6591, -21.4956) -> (-26.9299, -21.4956)
  line L516 (-26.9299, -21.4956) -> (-26.9299, -21.7664)
  line L517 (-26.9299, -21.7664) -> (-27.2008, -21.7664)
  line L518 (-27.2008, -21.7664) -> (-27.2008, -22.0373)
  line L519 (-27.2008, -22.0373) -> (-28.5549, -22.0373)
  line L520 (-28.5549, -22.0373) -> (-28.5549, -21.7664)
  line L521 (-28.5549, -21.7664) -> (-28.8258, -21.7664)
  line L522 (-28.8258, -21.7664) -> (-28.8258, -21.4956)
  line L523 (-28.8258, -21.4956) -> (-29.0966, -21.4956)
  line L524 (-29.0966, -21.4956) -> (-29.0966, -21.2248)
  line L525 (-29.0966, -21.2248) -> (-29.3674, -21.2248)
  line L526 (-29.3674, -21.2248) -> (-29.3674, -20.9539)
  line L527 (-29.3674, -20.9539) -> (-29.6383, -20.9539)
  line L528 (-29.6383, -20.9539) -> (-29.6383, -18.7873)
  line L529 (-29.6383, -18.7873) -> (-29.3674, -18.7873)
  line L530 (-29.3674, -18.7873) -> (-29.3674, -18.5164)
  line L531 (-29.3674, -18.5164) -> (-29.0966, -18.5164)
  line L532 (-29.0966, -18.5164) -> (-29.0966, -18.2456)
  line L533 (-29.0966, -18.2456) -> (-28.8258, -18.2456)
  line L534 (-28.8258, -18.2456) -> (-28.8258, -17.9748)
  line L535 (-28.8258, -17.9748) -> (-28.5549, -17.9748)
  line L536 (-28.5549, -17.9748) -> (-28.5549, -17.7039)
  line L537 (-28.5549, -17.7039) -> (-27.2008, -17.7039)
  line L538 (-23.4091, -17.7039) -> (-23.4091, -17.9748)
  line L539 (-23.4091, -17.9748) -> (-23.1383, -17.9748)
  line L540 (-23.1383, -17.9748) -> (-23.1383, -18.2456)
  line L541 (-23.1383, -18.2456) -> (-22.8674, -18.2456)
  line L542 (-22.8674, -18.2456) -> (-22.8674, -18.5164)
  line L543 (-22.8674, -18.5164) -> (-22.5966, -18.5164)
  line L544 (-22.5966, -18.5164) -> (-22.5966, -18.7873)
  line L545 (-22.5966, -18.7873) -> (-22.3258, -18.7873)
  line L546 (-22.3258, -18.7873) -> (-22.3258, -22.0373)
  line L547 (-22.3258, -22.0373) -> (-22.8674, -22.0373)
  line L548 (-22.8674, -22.0373) -> (-22.8674, -20.9539)
  line L549 (-22.8674, -20.9539) -> (-24.2216, -20.9539)
  line L550 (-24.2216, -20.9539) -> (-24.2216, -22.0373)
  line L551 (-24.2216, -22.0373) -> (-24.7633, -22.0373)
  line L552 (-24.7633, -22.0373) -> (-24.7633, -18.7873)
  line L553 (-24.7633, -18.7873) -> (-24.4924, -18.7873)
  line L554 (-24.4924, -18.7873) -> (-24.4924, -18.5164)
  line L555 (-24.4924, -18.5164) -> (-24.2216, -18.5164)
  line L556 (-24.2216, -18.5164) -> (-24.2216, -18.2456)
  line L557 (-24.2216, -18.2456) -> (-23.9508, -18.2456)
  line L558 (-23.9508, -18.2456) -> (-23.9508, -17.9748)
  line L559 (-23.9508, -17.9748) -> (-23.6799, -17.9748)
  line L560 (-23.6799, -17.9748) -> (-23.6799, -17.7039)
  line L561 (-23.6799, -17.7039) -> (-23.4091, -17.7039)
  line L562 (-19.3466, -17.7039) -> (-19.3466, -17.9748)
  line L563 (-19.3466, -17.9748) -> (-19.0758, -17.9748)
  line L564 (-19.0758, -17.9748) -> (-19.0758, -18.2456)
  line L565 (-19.0758, -18.2456) -> (-18.8049, -18.2456)
  line L566 (-18.8049, -18.2456) -> (-18.8049, -18.5164)
  line L567 (-18.8049, -18.5164) -> (-18.5341, -18.5164)
  line L568 (-18.5341, -18.5164) -> (-18.5341, -18.2456)
  line L569 (-18.5341, -18.2456) -> (-18.2633, -18.2456)
  line L570 (-18.2633, -18.2456) -> (-18.2633, -17.9748)
  line L571 (-18.2633, -17.9748) -> (-17.9924, -17.9748)
  line L572 (-17.9924, -17.9748) -> (-17.9924, -17.7039)
  line L573 (-17.9924, -17.7039) -> (-17.4508, -17.7039)
  line L574 (-17.4508, -17.7039) -> (-17.4508, -17.9748)
  line L575 (-17.4508, -17.9748) -> (-17.1799, -17.9748)
  line L576 (-17.1799, -17.9748) -> (-17.1799, -18.2456)
  line L577 (-17.1799, -18.2456) -> (-16.9091, -18.2456)
  line L578 (-16.9091, -18.2456) -> (-16.9091, -18.5164)
  line L579 (-16.9091, -18.5164) -> (-16.6383, -18.5164)
  line L580 (-16.6383, -18.5164) -> (-16.6383, -18.7873)
  line L581 (-16.6383, -18.7873) -> (-16.3674, -18.7873)
  line L582 (-16.3674, -18.7873) -> (-16.3674, -22.0373)
  line L583 (-16.3674, -22.0373) -> (-16.9091, -22.0373)
  line L584 (-16.9091, -22.0373) -> (-16.9091, -18.7873)
  line L585 (-16.9091, -18.7873) -> (-17.1799, -18.7873)
  line L586 (-17.1799, -18.7873) -> (-17.1799, -18.5164)
  line L587 (-17.1799, -18.5164) -> (-17.4508, -18.5164)
  line L588 (-17.4508, -18.5164) -> (-17.4508, -18.2456)
  line L589 (-17.4508, -18.2456) -> (-17.9924, -18.2456)
  line L590 (-17.9924, -18.2456) -> (-17.9924, -18.5164)
  line L591 (-17.9924, -18.5164) -> (-18.2633, -18.5164)
  line L592 (-18.2633, -18.5164) -> (-18.2633, -18.7873)
  line L593 (-18.2633, -18.7873) -> (-18.5341, -18.7873)
  line L594 (-18.5341, -18.7873) -> (-18.5341, -20.1414)
  line L595 (-18.5341, -20.1414) -> (-18.8049, -20.1414)
  line L596 (-18.8049, -20.1414) -> (-18.8049, -18.7873)
  line L597 (-18.8049, -18.7873) -> (-19.0758, -18.7873)
  line L598 (-19.0758, -18.7873) -> (-19.0758, -18.5164)
  line L599 (-19.0758, -18.5164) -> (-19.3466, -18.5164)
  line L600 (-19.3466, -18.5164) -> (-19.3466, -18.2456)
  line L601 (-19.3466, -18.2456) -> (-19.8883, -18.2456)
  line L602 (-19.8883, -18.2456) -> (-19.8883, -18.5164)
  line L603 (-19.8883, -18.5164) -> (-20.1591, -18.5164)
  line L604 (-20.1591, -18.5164) -> (-20.1591, -18.7873)
  line L605 (-20.1591, -18.7873) -> (-20.4299, -18.7873)
  line L606 (-20.4299, -18.7873) -> (-20.4299, -22.0373)
  line L607 (-20.4299, -22.0373) -> (-20.9716, -22.0373)
  line L608 (-20.9716, -22.0373) -> (-20.9716, -18.7873)
  line L609 (-20.9716, -18.7873) -> (-20.7008, -18.7873)
  line L610 (-20.7008, -18.7873) -> (-20.7008, -18.5164)
  line L611 (-20.7008, -18.5164) -> (-20.4299, -18.5164)
  line L612 (-20.4299, -18.5164) -> (-20.4299, -18.2456)
  line L613 (-20.4299, -18.2456) -> (-20.1591, -18.2456)
  line L614 (-20.1591, -18.2456) -> (-20.1591, -17.9748)
  line L615 (-20.1591, -17.9748) -> (-19.8883, -17.9748)
  line L616 (-19.8883, -17.9748) -> (-19.8883, -17.7039)
  line L617 (-19.8883, -17.7039) -> (-19.3466, -17.7039)
  line L618 (-12.5758, -17.7039) -> (-12.5758, -18.2456)
  line L619 (-12.5758, -18.2456) -> (-14.4716, -18.2456)
  line L620 (-14.4716, -18.2456) -> (-14.4716, -19.5998)
  line L621 (-14.4716, -19.5998) -> (-13.6591, -19.5998)
  line L622 (-13.6591, -19.5998) -> (-13.6591, -20.1414)
  line L623 (-13.6591, -20.1414) -> (-14.4716, -20.1414)
  line L624 (-14.4716, -20.1414) -> (-14.4716, -21.4956)
  line L625 (-14.4716, -21.4956) -> (-12.5758, -21.4956)
  line L626 (-12.5758, -21.4956) -> (-12.5758, -22.0373)
  line L627 (-12.5758, -22.0373) -> (-15.0133, -22.0373)
  line L628 (-15.0133, -22.0373) -> (-15.0133, -17.7039)
  line L629 (-15.0133, -17.7039) -> (-12.5758, -17.7039)
  line L630 (-7.7008, -17.7039) -> (-7.7008, -18.2456)
  line L631 (-7.7008, -18.2456) -> (-10.1383, -18.2456)
  line L632 (-10.1383, -18.2456) -> (-10.1383, -18.5164)
  line L633 (-10.1383, -18.5164) -> (-10.4091, -18.5164)
  line L634 (-10.4091, -18.5164) -> (-10.4091, -19.0581)
  line L635 (-10.4091, -19.0581) -> (-10.1383, -19.0581)
  line L636 (-10.1383, -19.0581) -> (-10.1383, -19.3289)
  line L637 (-10.1383, -19.3289) -> (-9.8674, -19.3289)
  line L638 (-9.8674, -19.3289) -> (-9.8674, -19.5998)
  line L639 (-9.8674, -19.5998) -> (-8.5133, -19.5998)
  line L640 (-8.5133, -19.5998) -> (-8.5133, -20.1414)
  line L641 (-8.5133, -20.1414) -> (-8.2424, -20.1414)
  line L642 (-8.2424, -20.1414) -> (-8.2424, -20.4123)
  line L643 (-8.2424, -20.4123) -> (-7.9716, -20.4123)
  line L644 (-7.9716, -20.4123) -> (-7.9716, -20.6831)
  line L645 (-7.9716, -20.6831) -> (-7.7008, -20.6831)
  line L646 (-7.7008, -20.6831) -> (-7.7008, -21.2248)
  line L647 (-7.7008, -21.2248) -> (-7.9716, -21.2248)
  line L648 (-7.9716, -21.2248) -> (-7.9716, -21.4956)
  line L649 (-7.9716, -21.4956) -> (-8.2424, -21.4956)
  line L650 (-8.2424, -21.4956) -> (-8.2424, -21.7664)
  line L651 (-8.2424, -21.7664) -> (-8.5133, -21.7664)
  line L652 (-8.5133, -21.7664) -> (-8.5133, -22.0373)
  line L653 (-8.5133, -22.0373) -> (-10.9508, -22.0373)
  line L654 (-10.9508, -22.0373) -> (-10.9508, -21.4956)
  line L655 (-10.9508, -21.4956) -> (-8.5133, -21.4956)
  line L656 (-8.5133, -21.4956) -> (-8.5133, -21.2248)
  line L657 (-8.5133, -21.2248) -> (-8.2424, -21.2248)
  line L658 (-8.2424, -21.2248) -> (-8.2424, -20.6831)
  line L659 (-8.2424, -20.6831) -> (-8.5133, -20.6831)
  line L660 (-8.5133, -20.6831) -> (-8.5133, -20.4123)
  line L661 (-8.5133, -20.4123) -> (-8.7841, -20.4123)
  line L662 (-8.7841, -20.4123) -> (-8.7841, -20.1414)
  line L663 (-8.7841, -20.1414) -> (-9.8674, -20.1414)
  line L664 (-9.8674, -20.1414) -> (-9.8674, -19.8706)
  line L665 (-9.8674, -19.8706) -> (-10.1383, -19.8706)
  line L666 (-10.1383, -19.8706) -> (-10.1383, -19.5998)
  line L667 (-10.1383, -19.5998) -> (-10.4091, -19.5998)
  line L668 (-10.4091, -19.5998) -> (-10.4091, -19.3289)
  line L669 (-10.4091, -19.3289) -> (-10.6799, -19.3289)
  line L670 (-10.6799, -19.3289) -> (-10.6799, -19.0581)
  line L671 (-10.6799, -19.0581) -> (-10.9508, -19.0581)
  line L672 (-10.9508, -19.0581) -> (-10.9508, -18.5164)
  line L673 (-10.9508, -18.5164) -> (-10.6799, -18.5164)
  line L674 (-10.6799, -18.5164) -> (-10.6799, -18.2456)
  line L675 (-10.6799, -18.2456) -> (-10.4091, -18.2456)
  line L676 (-10.4091, -18.2456) -> (-10.4091, -17.9748)
  line L677 (-10.4091, -17.9748) -> (-10.1383, -17.9748)
  line L678 (-10.1383, -17.9748) -> (-10.1383, -17.7039)
  line L679 (-10.1383, -17.7039) -> (-7.7008, -17.7039)
  line L680 (-23.6799, -18.2456) -> (-23.6799, -18.5164)
  line L681 (-23.6799, -18.5164) -> (-23.9508, -18.5164)
  line L682 (-23.9508, -18.5164) -> (-23.9508, -18.7873)
  line L683 (-23.9508, -18.7873) -> (-24.2216, -18.7873)
  line L684 (-24.2216, -18.7873) -> (-24.2216, -20.6831)
  line L685 (-24.2216, -20.6831) -> (-22.8674, -20.6831)
  line L686 (-22.8674, -20.6831) -> (-22.8674, -18.7873)
  line L687 (-22.8674, -18.7873) -> (-23.1383, -18.7873)
  line L688 (-23.1383, -18.7873) -> (-23.1383, -18.5164)
  line L689 (-23.1383, -18.5164) -> (-23.4091, -18.5164)
  line L690 (-23.4091, -18.5164) -> (-23.4091, -18.2456)
  line L691 (-23.4091, -18.2456) -> (-23.6799, -18.2456)
  line L692 (-23.4091, -18.7873) -> (-23.4091, -19.0581)
  line L693 (-23.4091, -19.0581) -> (-23.1383, -19.0581)
  line L694 (-23.1383, -19.0581) -> (-23.1383, -20.4123)
  line L695 (-23.1383, -20.4123) -> (-23.9508, -20.4123)
  line L696 (-23.9508, -20.4123) -> (-23.9508, -19.0581)
  line L697 (-23.9508, -19.0581) -> (-23.6799, -19.0581)
  line L698 (-23.6799, -19.0581) -> (-23.6799, -18.7873)
  line L699 (-23.6799, -18.7873) -> (-23.4091, -18.7873)